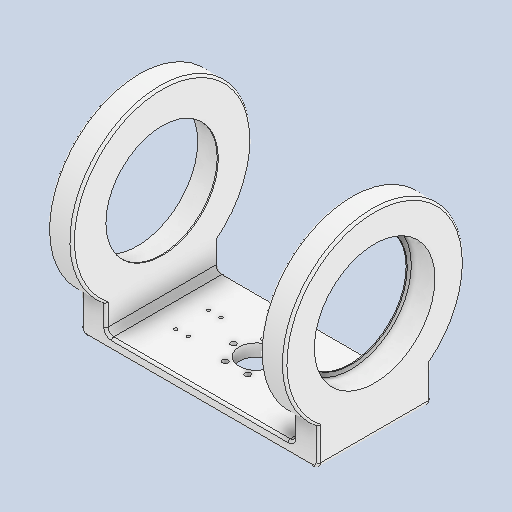
# Autodesk Inventor part: base
Saved by Autodesk Inventor 2025.3 (Build 293356030, 356C)
## iProperties
Created: 2025-08-30
Part Number: base
Material: PLA+ filament
Document SubType Name: Modeling
Designer: MSI
Density: 1.23 g/cm^3
Appearance: 일반
Mass: 915.953 g
Surface Area: 1301.23 cm^2
Volume: 744.677 cm^3
Author: MSI
Autodesk Inventor part; units mm, degrees
ref_plane "YZ Plane" through (0, 0, 0) normal (1, 0, 0) x (0, 1, 0)
ref_plane "XZ Plane" through (0, 0, 0) normal (0, 1, 0) x (-1, 0, 0)
ref_plane "XY Plane" through (0, 0, 0) normal (0, 0, 1) x (1, 0, 0)
sketch "스케치1" plane through (0, 0, 0) normal (1, 0, 0) x (0, 1, 0)
  circle A0 centre (0, 0) radius 80
  line L0 (0, 50) -> (-96, 50)
  line L1 (-96, 50) -> (-96, -50)
  line L2 (-96, -50) -> (0, -50)
  line L3 (0, -50) -> (0, 50)
  point P0 (-96, 0)
  point P1 (-62.45, -50)
  point P2 (-62.45, 50)
  dimension "d0" = 160
  dimension "d1" = 96
  dimension "d36" = 100
  constraints: 8 end point, 2 coincident, 2 midpoint, 2 parallel, 1 centre point, 1 horizontal, 1 horizontal alignment, 1 perpendicular
  measures "d0" diameter of A0
  measures "d1" distance of L1.end L2.end
  measures "d36" distance of L0.end L1.end
extrude "돌출1" add sketch "스케치1" along normal mid plane 211
sketch "스케치2" plane through (0, 0, 0) normal (0, 0, 1) x (1, 0, 0)
  line L0 (-105.5, 80) -> (105.5, 80) projected
  line L1 (-83.5, 80) -> (83.5, 80)
  line L2 (83.5, 80) -> (83.5, -86)
  line L3 (83.5, -86) -> (-83.5, -86)
  line L4 (-83.5, -86) -> (-83.5, 80)
  line L5 (-105.5, -96) -> (105.5, -96) projected
  line L6 (105.5, -96) -> (105.5, -62.45) projected
  point P0 (0, 0)
  point P1 (0, -86)
  dimension "d4" = 10
  dimension "d5" = 22
  constraints: 8 end point, 2 parallel, 1 horizontal, 1 midpoint, 1 perpendicular, 1 point on line, 1 vertical alignment
  measures "d4" distance between parallel lines of L5 L3
  measures "d5" distance between parallel lines of L6 L2
extrude "돌출2" cut sketch "스케치2" along normal through all both and the other way through all
sketch "스케치3" plane through (-83.5, -86, -50) normal (0, 1, 0) x (1, 0, 0)
  point P0 (83.5, -50)
  point P1 (83.5, -50)
  constraints: 1 coincident
hole "구멍1" at (0, -86, 0) direction (0, -1, 0) diameter 30 end through all
sketch "스케치4" plane through (105.5, 0, 0) normal (1, 0, 0) x (0, 0, -1)
  arc A0 (50, -62.45) -> (-50, -62.45) centre (0, 0) ccw projected
  point P0 (-80, 0)
  constraints: 1 coincident
hole "구멍2" at (105.5, 0, 0) direction (-1, 0, 0) diameter 100 end through all counterbore diameter 107.25 counterbore depth 21
mirror "미러1" about plane through (0, 0, 0) normal (1, 0, 0) of "구멍2"
fillet "모깎기1" radius 5 2 edges at (-83.5, -86, 0) (83.5, -86, 0)
fillet "모깎기2" radius 5 2 edges at (105.5, -96, 0) (-105.5, -96, 0)
fillet "모깎기3" radius 2 24 edges at (-83.5, 80, 0) (-83.5, -71.725, -50) (-82.0355, -84.5355, -50) (0, -86, -50) (82.0355, -84.5355, -50) (83.5, -71.725, -50) (83.5, 80, 0) (83.5, -71.725, 50) (82.0355, -84.5355, 50) (0, -86, 50) (-82.0355, -84.5355, 50) (-83.5, -71.725, 50) (-105.5, 80, 0) (-105.5, -76.725, -50) (-104.0355, -94.5355, -50) (0, -96, -50) (104.0355, -94.5355, -50) (105.5, -76.725, -50) (105.5, 80, 0) (105.5, -76.725, 50) (104.0355, -94.5355, 50) (0, -96, 50) (-104.0355, -94.5355, 50) (-105.5, -76.725, 50)
sketch "스케치8" plane through (-100.5, -96, 48) normal (0, -1, 0) x (1, 0, 0)
  circle A0 centre (100.5, -48) radius 40
  circle A1 centre (100.5, -48) radius 15 projected
  dimension "d56" = 80
  constraints: 1 centre point, 1 coincident
  measures "d56" diameter of A0
extrude "돌출3" add sketch "스케치8" along normal blind 1
sketch "스케치5" plane through (-78.5, -86, -48) normal (0, 1, 0) x (1, 0, 0)
  line L0 (78.5, -48) -> (58.5, -48) construction
  dimension "d25" = 20
  constraints: 2 end point, 1 horizontal
  measures "d25" distance of L0.start L0.end
hole "구멍3" at (-20, -86, 0) direction (0, -1, 0) diameter 5 end through all
pattern_circular "원형 패턴1" count 6 over 360 about axis through (0, -403.9575, 0) along (0, 1, 0) of "구멍3"
sketch "스케치6" plane through (-78.5, -86, -48) normal (0, 1, 0) x (1, 0, 0)
  line L0 (19.721, -31.5) -> (34.721, -31.5)
  line L1 (34.721, -31.5) -> (34.721, -64.5)
  line L2 (34.721, -64.5) -> (19.721, -64.5)
  line L3 (19.721, -64.5) -> (19.721, -31.5)
  line L4 (19.721, -31.5) -> (34.721, -64.5) construction
  line L5 (34.721, -31.5) -> (19.721, -64.5) construction
  circle A0 centre (78.5, -48) radius 15 projected
  line L6 (78.5, -33) -> (78.5, -63) construction
  line L7 (137.279, -31.5) -> (122.279, -31.5)
  line L8 (122.279, -31.5) -> (122.279, -64.5)
  line L9 (122.279, -64.5) -> (137.279, -64.5)
  line L10 (137.279, -64.5) -> (137.279, -31.5)
  line L11 (137.279, -31.5) -> (122.279, -64.5) construction
  line L12 (122.279, -31.5) -> (137.279, -64.5) construction
  line L13 (32.721, -62.5) -> (32.721, -33.5)
  line L14 (32.721, -33.5) -> (21.721, -33.5)
  line L15 (21.721, -33.5) -> (21.721, -62.5)
  line L16 (21.721, -62.5) -> (32.721, -62.5)
  line L17 (135.279, -62.5) -> (124.279, -62.5)
  line L18 (124.279, -62.5) -> (124.279, -33.5)
  line L19 (124.279, -33.5) -> (135.279, -33.5)
  line L20 (135.279, -33.5) -> (135.279, -62.5)
  point P0 (27.221, -48)
  point P1 (129.779, -48)
  dimension "d37" = 43.779
  dimension "d38" = 15
  dimension "d39" = 33
  dimension "d47" = 2
  dimension "d48" = 2
  constraints: 42 end point, 5 symmetric about line, 4 parallel, 3 midpoint, 2 perpendicular, 2 point on circle, 1 coincident, 1 horizontal, 1 horizontal alignment, 1 vertical, 6 other
  measures "d37" distance from line of point (78.5, -48) L1
  measures "d38" distance of L1.end L2.end
  measures "d39" distance of L2.end L0.start
  measures "d47" distance between parallel lines of L1 L13
  measures "d48" distance between parallel lines of L9 L17
hole "구멍4" at (45.779, -86, 14.5) at (45.779, -86, -14.5) at (56.779, -86, -14.5) at (56.779, -86, 14.5) at (-45.779, -86, -14.5) at (-45.779, -86, 14.5) at (-56.779, -86, 14.5) at (-56.779, -86, -14.5) direction (0, -1, 0) diameter 2.9 end through all clearance for "Flat Head Machine Screw" size "M2.5" standard "Ansi Metric M Profile"
